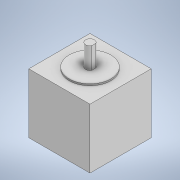
# Autodesk Inventor part: Linear Rail motor
Saved by Autodesk Inventor 2022 (Build 260153000, 153)
## iProperties
Created: 2021-11-30
Part Number: Linear Rail motor
Material: Generic
Document SubType Name: Modeling
Designer: efred
Density: 1 g/cm^3
Appearance: Default
Author: efred
Autodesk Inventor part; units mm, degrees
ref_plane "YZ Plane" through (0, 0, 0) normal (1, 0, 0) x (0, 1, 0)
ref_plane "XZ Plane" through (0, 0, 0) normal (0, 1, 0) x (-1, 0, 0)
ref_plane "XY Plane" through (0, 0, 0) normal (0, 0, 1) x (1, 0, 0)
sketch "Sketch1" plane through (0, 0, 0) normal (0, 1, 0) x (-1, 0, 0)
  line L0 (-28, 28) -> (28, 28)
  line L1 (28, 28) -> (28, -28)
  line L2 (28, -28) -> (-28, -28)
  line L3 (-28, -28) -> (-28, 28)
  line L4 (-28, 28) -> (28, -28) construction
  line L5 (28, 28) -> (-28, -28) construction
  point P0 (0, 0)
  dimension "d0" = 56
  dimension "d1" = 56
  constraints: 12 end point, 2 midpoint, 2 parallel, 1 horizontal, 1 perpendicular
  measures "d0" distance of L1.end L2.end
  measures "d1" distance of L0.end L1.end
extrude "Extrusion1" add sketch "Sketch1" along normal blind 54.6
sketch "Sketch2" plane through (0, 54.6, 0) normal (0, 1, 0) x (1, 0, 0)
  circle A0 centre (0, 0) radius 19
  dimension "d4" = 38
  constraints: 1 centre point, 1 coincident
  measures "d4" diameter of A0
extrude "Extrusion2" add sketch "Sketch2" along normal blind 1.5
sketch "Sketch3" plane through (0, 56.1, 0) normal (0, 1, 0) x (1, 0, 0)
  arc A0 (3.5, 1.9365) -> (3.5, -1.9365) centre (0, 0) ccw
  line L0 (3.5, -1.9365) -> (3.5, 1.9365)
  point P0 (4, 0)
  dimension "d7" = 8
  dimension "d8" = 0.5
  constraints: 3 point on circle, 2 end point, 1 centre point, 1 coincident, 1 horizontal alignment, 1 vertical
  measures "d7" diameter of A0
  measures "d8" distance from line of point (4, 0) L0
extrude "Extrusion3" add sketch "Sketch3" along normal blind 19.5
body "Solid1"
